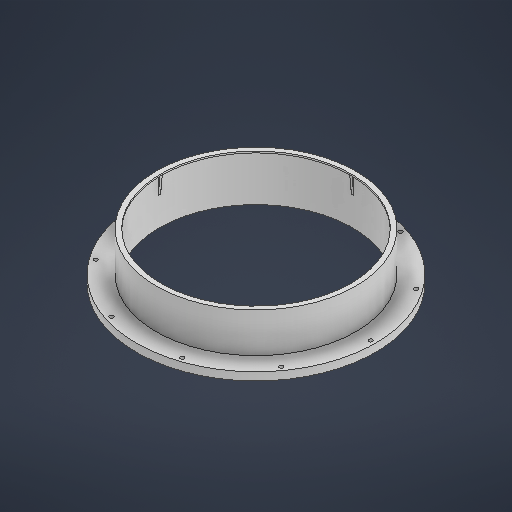
# Autodesk Inventor part: Cylinder Replacement- 01
Saved by Autodesk Inventor 2025 (Build 290162000, 162)
## iProperties
Created: 2024-04-11
Part Number: Cylinder Replacement- 01
Material: Generic
Document SubType Name: Modeling
Designer: Thienan Hoang
Density: 1 g/cm^3
Appearance: Default
Author: Thienan Hoang
Autodesk Inventor part; units mm, degrees
ref_plane "YZ Plane" through (0, 0, 0) normal (1, 0, 0) x (0, 1, 0)
ref_plane "XZ Plane" through (0, 0, 0) normal (0, 1, 0) x (-1, 0, 0)
ref_plane "XY Plane" through (0, 0, 0) normal (0, 0, 1) x (1, 0, 0)
sketch "Sketch1" plane through (0, 0, 0) normal (0, 1, 0) x (-1, 0, 0)
  circle A0 centre (0, 0) radius 151
  circle A1 centre (0, 0) radius 126
  circle A2 centre (0, 0) radius 122
  dimension "Absolute_Diameter" = 302
  dimension "Diameter_No_Outer_Lip" = 252
  dimension "Inner_Cylinder_Diameter" = 244
  constraints: 3 centre point, 3 coincident
  measures "Absolute_Diameter" diameter of A0
  measures "Diameter_No_Outer_Lip" diameter of A1
  measures "Inner_Cylinder_Diameter" diameter of A2
extrude "Extrusion1" add sketch "Sketch1" along normal blind 10 contours A0
extrude "Extrusion2" add sketch "Sketch1" along normal blind 60 contours A1
sketch "Sketch2" plane through (0, 60, 0) normal (0, 1, 0) x (1, 0, 0)
  circle A0 centre (0, 0) radius 120
  circle A1 centre (0, 0) radius 126
  dimension "Lip_Diameter_Out" = 240
  dimension "Top_Outer_Lip_Diameter" = 252
  constraints: 2 centre point, 2 coincident
  measures "Lip_Diameter_Out" diameter of A0
  measures "Top_Outer_Lip_Diameter" diameter of A1
extrude "Extrusion7" add sketch "Sketch2" against normal blind 2
ref_plane "Work Plane2" through (0, 10, 0) normal (0, 1, 0) x (1, 0, 0)
sketch "Sketch3" plane through (0, 10, 0) normal (0, 1, 0) x (1, 0, 0)
  circle A0 centre (0, 0) radius 145
  circle A1 centre (-145, 0) radius 2.5
  circle A2 centre (-117.3075, -85.2289) radius 2.5
  circle A3 centre (-44.8075, -137.9032) radius 2.5
  circle A4 centre (44.8075, -137.9032) radius 2.5
  circle A5 centre (117.3075, -85.2289) radius 2.5
  circle A6 centre (145, 0) radius 2.5
  circle A7 centre (117.3075, 85.2289) radius 2.5
  circle A8 centre (44.8075, 137.9032) radius 2.5
  circle A9 centre (-44.8075, 137.9032) radius 2.5
  circle A10 centre (-117.3075, 85.2289) radius 2.5
  dimension "d27" = 290
  dimension "d28" = 5
  dimension "d31" = 360
  constraints: 10 centre point, 1 coincident, 1 horizontal alignment, 23 other
  measures "d28" diameter of A1
extrude "Extrusion8" cut sketch "Sketch3" against normal blind 10 contours A0 A6 | A0 A6 | A7 A0 | A0 A7 | A5 A0 | A0 A5 | A8 A0 | A0 A8 | A4 A0 | A0 A4 | A9 A0 | A0 A9 | A3 A0 | A0 A3 | A10 A0 | A0 A10 | A2 A0 | A0 A2 | A1 A0 | A0 A1
sketch "Sketch24" plane through (0, 60, 0) normal (0, 1, 0) x (1, 0, 0)
  circle A0 centre (0, 0) radius 51
  circle A1 centre (0, -51) radius 2.75
  circle A2 centre (44.1673, -25.5) radius 2.75
  circle A3 centre (44.1673, 25.5) radius 2.75
  circle A4 centre (0, 51) radius 2.75
  circle A5 centre (-44.1673, 25.5) radius 2.75
  circle A6 centre (-44.1673, -25.5) radius 2.75
  dimension "d230" = 102
  dimension "d231" = 5.5
  dimension "d234" = 360
  constraints: 6 centre point, 1 coincident, 1 vertical alignment, 15 other
  measures "d231" diameter of A1
extrude "Extrusion30" [suppressed]
sketch "Sketch26" plane through (0, 0, 0) normal (1, 0, 0) x (0, 1, 0)
  line L0 (2, 63) -> (23.9089, 61)
  line L1 (2, -63) -> (23.9089, -61)
  point P0 (0, 0)
  dimension "d239" = 22
  dimension "d240" = 22
  constraints: 4 end point
  measures "d239" distance of L0.start L0.end
  measures "d240" distance of L1.start L1.end
feature "Rib2" [suppressed]
feature "Rib3" [suppressed]
sketch "Sketch27" plane through (0, 0, 0) normal (0, 0, 1) x (1, 0, 0)
  line L0 (63, 2) -> (61, 23.9089)
  line L1 (-63, 2) -> (-61, 23.9089)
  point P0 (0, 0)
  dimension "d259" = 22
  dimension "d260" = 22
  constraints: 4 end point
  measures "d259" distance of L0.start L0.end
  measures "d260" distance of L1.start L1.end
feature "Rib4" [suppressed]
feature "Rib5" [suppressed]
sketch "Sketch28" plane through (0, 0, 0) normal (1, 0, 0) x (0, 1, 0)
  line L0 (60, 0) -> (0, 0)
  line L1 (58, 61.4891) -> (36.0921, 63.5)
  line L2 (2, 69.5) -> (23.9089, 67.5)
  line L3 (58, -61.4891) -> (36.0921, -63.5)
  line L4 (2, -69.5) -> (23.9089, -67.5)
  dimension "d274" = 22
  dimension "d275" = 22
  constraints: 10 end point, 4 symmetric about line
  measures "d274" distance of L1.start L1.end
  measures "d275" distance of L2.start L2.end
feature "Rib6" [suppressed]
feature "Rib7" [suppressed]
sketch "Sketch29" plane through (0, 0, 0) normal (0, 0, 1) x (1, 0, 0)
  line L0 (0, 60) -> (0, 0.6462)
  line L1 (61.5, 58) -> (63.5, 36.0911)
  line L2 (69.5, 2) -> (67.5, 23.9089)
  line L3 (-61.5, 58) -> (-63.5, 36.0911)
  line L4 (-69.5, 2) -> (-67.5, 23.9089)
  point P0 (0, 0)
  dimension "d288" = 22
  dimension "d289" = 22
  constraints: 10 end point, 4 symmetric about line, 1 vertical
  measures "d288" distance of L1.start L1.end
  measures "d289" distance of L2.start L2.end
feature "Rib8" [suppressed]
feature "Rib9" [suppressed]
sketch "Sketch30" plane through (0, 0, 0) normal (1, 0, 0) x (0, 1, 0)
  line L0 (58, 0) -> (0, 0)
  line L1 (58, -68) -> (36.0911, -70)
  line L2 (2, -76) -> (23.9089, -74)
  line L3 (58, 68) -> (36.0911, 70)
  line L4 (2, 76) -> (23.9089, 74)
  dimension "d302" = 22
  dimension "d303" = 22
  constraints: 10 end point, 4 symmetric about line, 1 horizontal
  measures "d302" distance of L1.start L1.end
  measures "d303" distance of L2.start L2.end
feature "Rib10" [suppressed]
feature "Rib11" [suppressed]
sketch "Sketch31" plane through (0, 0, 0) normal (0, 0, 1) x (1, 0, 0)
  line L0 (0, 60) -> (0, 0)
  line L1 (-68, 58) -> (-70, 36.0911)
  line L2 (-76, 2) -> (-74, 23.9089)
  line L3 (68, 58) -> (70, 36.0911)
  line L4 (76, 2) -> (74, 23.9089)
  dimension "d316" = 22
  dimension "d317" = 22
  constraints: 10 end point, 4 symmetric about line, 1 vertical
  measures "d316" distance of L1.start L1.end
  measures "d317" distance of L2.start L2.end
feature "Rib12" [suppressed]
feature "Rib13" [suppressed]
sketch "Sketch32" plane through (0, 0, 0) normal (0, 0, 1) x (1, 0, 0)
  line L0 (0, 58) -> (0, 0)
  line L1 (-74.6125, 58) -> (-76.5, 36.0811)
  line L2 (-82.5, 2) -> (-80.5, 23.9089)
  line L3 (74.6125, 58) -> (76.5, 36.0811)
  line L4 (82.5, 2) -> (80.5, 23.9089)
  dimension "d330" = 22
  dimension "d331" = 22
  constraints: 10 end point, 4 symmetric about line, 1 vertical
  measures "d330" distance of L1.start L1.end
  measures "d331" distance of L2.start L2.end
feature "Rib14" [suppressed]
feature "Rib15" [suppressed]
sketch "Sketch33" plane through (0, 0, 0) normal (1, 0, 0) x (0, 1, 0)
  line L0 (60, 0) -> (0, 0)
  line L1 (58, 74.5) -> (36.0911, 76.5)
  line L2 (2, 82.5) -> (23.9089, 80.5)
  line L3 (58, -74.5) -> (36.0911, -76.5)
  line L4 (2, -82.5) -> (23.9089, -80.5)
  dimension "d344" = 22
  dimension "d345" = 22
  constraints: 10 end point, 4 symmetric about line, 1 horizontal
  measures "d344" distance of L1.start L1.end
  measures "d345" distance of L2.start L2.end
feature "Rib16" [suppressed]
feature "Rib17" [suppressed]
sketch "Sketch34" plane through (0, 0, 0) normal (1, 0, 0) x (0, 1, 0)
  line L0 (60, 0) -> (0, 0)
  line L1 (58, 80.9625) -> (36.0946, 83)
  line L2 (2, 89) -> (23.9089, 87)
  line L3 (58, -80.9625) -> (36.0946, -83)
  line L4 (2, -89) -> (23.9089, -87)
  dimension "d358" = 22
  dimension "d359" = 22
  constraints: 10 end point, 4 symmetric about line, 1 horizontal
  measures "d358" distance of L1.start L1.end
  measures "d359" distance of L2.start L2.end
feature "Rib18" [suppressed]
feature "Rib19" [suppressed]
sketch "Sketch35" plane through (0, 0, 0) normal (0, 0, 1) x (1, 0, 0)
  line L0 (0, 60) -> (0, 0)
  line L1 (80.9625, 58) -> (83, 36.0946)
  line L2 (89, 2) -> (87, 23.9089)
  line L3 (-80.9625, 58) -> (-83, 36.0946)
  line L4 (-89, 2) -> (-87, 23.9089)
  dimension "d372" = 22
  dimension "d373" = 22
  constraints: 10 end point, 4 symmetric about line, 1 vertical
  measures "d372" distance of L1.start L1.end
  measures "d373" distance of L2.start L2.end
feature "Rib20" [suppressed]
feature "Rib21" [suppressed]
sketch "Sketch36" plane through (0, 0, 0) normal (0, 0, 1) x (1, 0, 0)
  line L0 (0, 58) -> (0, 0)
  line L1 (87.5, 58) -> (89.5, 36.0911)
  line L2 (95.5, 2) -> (93.5, 23.9089)
  line L3 (-87.5, 58) -> (-89.5, 36.0911)
  line L4 (-95.5, 2) -> (-93.5, 23.9089)
  dimension "d386" = 22
  dimension "d387" = 22
  constraints: 10 end point, 4 symmetric about line, 1 vertical
  measures "d386" distance of L1.start L1.end
  measures "d387" distance of L2.start L2.end
feature "Rib22" [suppressed]
feature "Rib23" [suppressed]
sketch "Sketch37" plane through (0, 0, 0) normal (1, 0, 0) x (0, 1, 0)
  line L0 (60.325, 0) -> (0, 0)
  line L1 (58, -87.5) -> (36.0911, -89.5)
  line L2 (2, -95.5) -> (23.9089, -93.5)
  line L3 (58, 87.5) -> (36.0911, 89.5)
  line L4 (2, 95.5) -> (23.9089, 93.5)
  dimension "d401" = 22
  constraints: 10 end point, 4 symmetric about line
  measures "d401" distance of L2.start L2.end
feature "Rib24" [suppressed]
feature "Rib25" [suppressed]
sketch "Sketch38" plane through (0, 0, 0) normal (0, 0, 1) x (1, 0, 0)
  line L0 (0, 60) -> (0, 0)
  line L1 (-94, 58) -> (-96, 36.0911)
  line L2 (-102, 2) -> (-100, 23.9089)
  line L3 (94, 58) -> (96, 36.0911)
  line L4 (102, 2) -> (100, 23.9089)
  dimension "d414" = 22
  dimension "d415" = 22
  constraints: 10 end point, 4 symmetric about line, 1 vertical
  measures "d414" distance of L1.start L1.end
  measures "d415" distance of L2.start L2.end
feature "Rib26" [suppressed]
feature "Rib27" [suppressed]
sketch "Sketch39" plane through (0, 0, 0) normal (1, 0, 0) x (0, 1, 0)
  line L0 (60, 0) -> (0, 0)
  line L1 (58, 94) -> (36.0911, 96)
  line L2 (2, 102) -> (23.9089, 100)
  line L3 (58, -94) -> (36.0911, -96)
  line L4 (2, -102) -> (23.9089, -100)
  dimension "d428" = 22
  dimension "d429" = 22
  constraints: 10 end point, 4 symmetric about line, 1 horizontal
  measures "d428" distance of L1.start L1.end
  measures "d429" distance of L2.start L2.end
feature "Rib28" [suppressed]
feature "Rib29" [suppressed]
sketch "Sketch40" plane through (0, 0, 0) normal (1, 0, 0) x (0, 1, 0)
  line L0 (60, 0) -> (0, 0)
  line L1 (58, 100.5) -> (36.0911, 102.5)
  line L2 (2, 108.5) -> (23.9089, 106.5)
  line L3 (58, -100.5) -> (36.0911, -102.5)
  line L4 (2, -108.5) -> (23.9089, -106.5)
  dimension "d442" = 22
  dimension "d443" = 22
  constraints: 10 end point, 4 symmetric about line, 1 horizontal
  measures "d442" distance of L1.start L1.end
  measures "d443" distance of L2.start L2.end
feature "Rib30" [suppressed]
feature "Rib31" [suppressed]
sketch "Sketch41" plane through (0, 0, 0) normal (0, 0, 1) x (1, 0, 0)
  line L0 (0, 60) -> (0, 0)
  line L1 (100.5, 58) -> (102.5, 36.0911)
  line L2 (108.5, 2) -> (106.5, 23.9089)
  line L3 (-100.5, 58) -> (-102.5, 36.0911)
  line L4 (-108.5, 2) -> (-106.5, 23.9089)
  dimension "d456" = 22
  dimension "d457" = 22
  constraints: 10 end point, 4 symmetric about line, 1 vertical
  measures "d456" distance of L1.start L1.end
  measures "d457" distance of L2.start L2.end
feature "Rib32" [suppressed]
feature "Rib33" [suppressed]
sketch "Sketch42" plane through (0, 0, 0) normal (1, 0, 0) x (0, 1, 0)
  line L0 (60, 0) -> (0, 0)
  line L1 (58, -107) -> (36.0911, -109)
  line L2 (2, -115) -> (23.9089, -113)
  line L3 (58, 107) -> (36.0911, 109)
  line L4 (2, 115) -> (23.9089, 113)
  dimension "d470" = 22
  dimension "d471" = 22
  constraints: 10 end point, 4 symmetric about line
  measures "d470" distance of L1.start L1.end
  measures "d471" distance of L2.start L2.end
feature "Rib34" [suppressed]
feature "Rib35" [suppressed]
sketch "Sketch43" plane through (0, 0, 0) normal (0, 0, 1) x (1, 0, 0)
  line L0 (0, 60) -> (0, 0)
  line L1 (-107, 58) -> (-109, 36.0911)
  line L2 (-115, 2) -> (-113, 23.9089)
  line L3 (107, 58) -> (109, 36.0911)
  line L4 (115, 2) -> (113, 23.9089)
  dimension "d484" = 22
  dimension "d485" = 22
  constraints: 10 end point, 4 symmetric about line
  measures "d484" distance of L1.start L1.end
  measures "d485" distance of L2.start L2.end
feature "Rib36" [suppressed]
feature "Rib37" [suppressed]
sketch "Sketch44" plane through (0, 0, 0) normal (0, 0, 1) x (1, 0, 0)
  line L0 (0, 60) -> (0, 0)
  line L1 (-113.5, 58) -> (-115.5, 36.0911)
  line L2 (-121.5, 2) -> (-119.5, 23.9089)
  line L3 (113.5, 58) -> (115.5, 36.0911)
  line L4 (121.5, 2) -> (119.5, 23.9089)
  dimension "d498" = 22
  dimension "d499" = 22
  constraints: 10 end point, 4 symmetric about line, 1 vertical
  measures "d498" distance of L1.start L1.end
  measures "d499" distance of L2.start L2.end
feature "Rib38" [suppressed]
feature "Rib39" [suppressed]
sketch "Sketch45" plane through (0, 0, 0) normal (1, 0, 0) x (0, 1, 0)
  line L0 (60, 0) -> (0, 0)
  line L1 (58, -113.5) -> (36.0911, -115.5)
  line L2 (2, -121.5) -> (23.9089, -119.5)
  line L3 (58, 113.5) -> (36.0911, 115.5)
  line L4 (2, 121.5) -> (23.9089, 119.5)
  dimension "d512" = 22
  dimension "d513" = 22
  constraints: 10 end point, 4 symmetric about line, 1 horizontal
  measures "d512" distance of L1.start L1.end
  measures "d513" distance of L2.start L2.end
feature "Rib40" [suppressed]
feature "Rib41" [suppressed]
sketch "Sketch46" plane through (0, 0, 0) normal (1, 0, 0) x (0, 1, 0)
  line L0 (60, 0) -> (0, 0)
  line L1 (58, -120) -> (36.0911, -122)
  line L2 (58, 120) -> (36.0911, 122)
  dimension "d526" = 22
  constraints: 6 end point, 2 symmetric about line
  measures "d526" distance of L1.start L1.end
extrude "Rib42" add sketch "Sketch46" along normal mid plane 3 rib yes fills toward (47.0501, -121.0498) open curves L1
extrude "Rib43" add sketch "Sketch46" along normal mid plane 3 rib yes fills toward (47.0501, 121.0498) open curves L2
sketch "Sketch47" plane through (0, 0, 0) normal (0, 0, 1) x (1, 0, 0)
  line L0 (0, 60) -> (0, 0)
  line L1 (-120, 58) -> (-122, 36.0911)
  line L2 (120, 58) -> (122, 36.0911)
  dimension "d539" = 22
  constraints: 6 end point, 2 symmetric about line, 1 vertical
  measures "d539" distance of L1.start L1.end
extrude "Rib44" add sketch "Sketch47" along normal mid plane 3 rib yes fills toward (-121.0498, 47.0501) open curves L1
extrude "Rib45" add sketch "Sketch47" along normal mid plane 3 rib yes fills toward (121.0498, 47.0501) open curves L2
body "Solid1"
